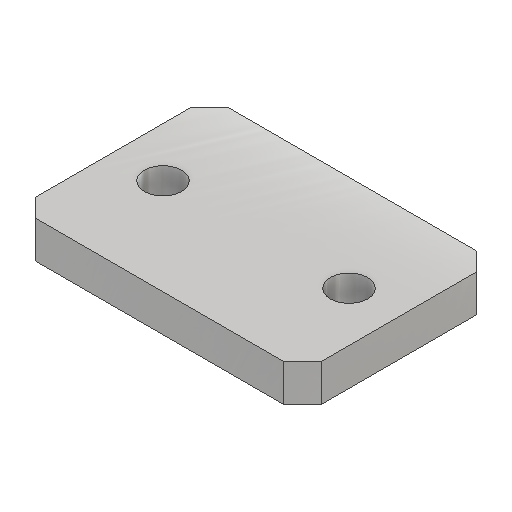
# Autodesk Inventor part: LC_ALU_3mm_Timing_Belt_Clamp_Y_Axis
Saved by Autodesk Inventor 2026.1 (Build 301233000, 233)
## iProperties
Created: 2016-06-19
Part Number: LC_ALU_3mm_Timing_Belt_Clamp_Y_Axis
Material: Ogólny
Document SubType Name: Modeling
Designer: Andrzej
Density: 1 g/cm^3
Appearance: Obrobione - aluminium
Mass: 1.01359 g
Surface Area: 9.5273 cm^2
Volume: 1.01359 cm^3
Author: Andrzej
Autodesk Inventor part; units mm, degrees
ref_plane "YZ Plane" through (0, 0, 0) normal (1, 0, 0) x (0, 1, 0)
ref_plane "XZ Plane" through (0, 0, 0) normal (0, 1, 0) x (-1, 0, 0)
ref_plane "XY Plane" through (0, 0, 0) normal (0, 0, 1) x (1, 0, 0)
sketch "Szkic1" plane through (0, 0, 0) normal (0, 0, 1) x (1, 0, 0)
  line L0 (-10.326, 7.3757) -> (12.674, 7.3757)
  line L1 (12.674, 7.3757) -> (12.674, -8.1243)
  line L2 (12.674, -8.1243) -> (-10.326, -8.1243)
  line L3 (-10.326, -8.1243) -> (-10.326, 7.3757)
  point P0 (0, 0)
  point P1 (-6.326, -0.3743)
  point P2 (8.674, -0.3743)
  dimension "d0" = 23
  dimension "d1" = 15.5
  dimension "d4" = 7.75
  dimension "d5" = 7.75
  dimension "d6" = 4
  dimension "d7" = 4
  constraints: 8 end point, 2 parallel, 1 horizontal, 1 perpendicular
  measures "d0" distance of L1.end L2.end
  measures "d1" distance of L0.end L1.end
  measures "d4" distance from line of L0 point (-6.326, -0.374)
  measures "d5" distance from line of L0 point (8.674, -0.374)
  measures "d6" distance from line of L3 point (-6.326, -0.374)
  measures "d7" distance from line of L1 point (8.674, -0.374)
extrude "Wyciągnięcie proste1" add sketch "Szkic1" along normal blind 3
hole "Otwór1" at (-6.326, -0.3743, 0) at (8.674, -0.3743, 0) direction (0, 0, 1) diameter 3 end through all
chamfer "Faza1" distance 1.5 angle 45 4 edges at (12.674, -8.1243, 1.5) (-10.326, -8.1243, 1.5) (-10.326, 7.3757, 1.5) (12.674, 7.3757, 1.5)
equation "\"d4\" = 0.5 * d1"
equation "\"d5\" = d4"
equation "\"d7\" = d6"
